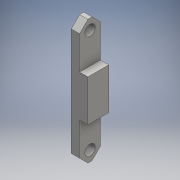
# Autodesk Inventor part: promo_arm2
Saved by Autodesk Inventor 2016 (Build 200138000, 138)
## iProperties
Created: 2016-05-12
Part Number: promo_arm2
Material: 一般
Document SubType Name: Modeling
Designer: 宏太
Density: 1 g/cm^3
Appearance: 既定
Mass: 0.364365 g
Surface Area: 4.86408 cm^2
Volume: 0.364365 cm^3
Author: 宏太
Autodesk Inventor part; units mm, degrees
ref_plane "YZ Plane" through (0, 0, 0) normal (1, 0, 0) x (0, 1, 0)
ref_plane "XZ Plane" through (0, 0, 0) normal (0, 1, 0) x (-1, 0, 0)
ref_plane "XY Plane" through (0, 0, 0) normal (0, 0, 1) x (1, 0, 0)
sketch "スケッチ1" plane through (0, 0, 0) normal (0, 1, 0) x (-1, 0, 0)
  line L0 (-2, -15) -> (2, -15)
  line L1 (2, -15) -> (2, 15)
  line L2 (2, 15) -> (-2, 15)
  line L3 (-2, 15) -> (-2, -15)
  line L4 (-2, -15) -> (2, 15) construction
  line L5 (2, -15) -> (-2, 15) construction
  point P0 (0, 0)
  dimension "d0" = 4
  dimension "d1" = 30
  constraints: 12 end point, 2 midpoint, 2 parallel, 1 horizontal, 1 perpendicular
  measures "d0" distance of L2.end L1.end
  measures "d1" distance of L1.end L0.end
extrude "押し出し1" add sketch "スケッチ1" along normal mid plane 5
sketch "スケッチ2" plane through (0, 2.5, 0) normal (0, 1, 0) x (1, 0, 0)
  line L0 (-2, -15) -> (2, -15) projected
  line L1 (0, -15) -> (2, -15)
  line L2 (2, -15) -> (2, -5)
  line L3 (2, -5) -> (0, -5)
  line L4 (0, -5) -> (0, -15)
  point P0 (0, 0)
  dimension "d4" = 2
  dimension "d5" = 10
  constraints: 8 end point, 2 parallel, 1 horizontal, 1 midpoint, 1 perpendicular
  measures "d4" distance of L3.end L2.end
  measures "d5" distance of L2.end L1.end
extrude "押し出し2" cut sketch "スケッチ2" against normal blind 5
sketch "スケッチ4" plane through (0, 2.5, 15) normal (1, 0, 0) x (0, 0, -1)
  circle A0 centre (2.5, -2.5) radius 1.25
  point P0 (15, -2.5)
  dimension "d12" = 2.5
  constraints: 1 centre point
  measures "d12" diameter of A0
extrude "押し出し4" cut sketch "スケッチ4" against normal blind 5
ref_plane "作業平面1" through (0, 2.5, -15) normal (-1, 0, 0) x (0, 0, 1)
sketch "スケッチ5" plane through (0, 2.5, -15) normal (-1, 0, 0) x (0, 0, 1)
  circle A0 centre (2.5, -2.5) radius 1.25
  point P0 (15, -2.5)
  dimension "d15" = 2.5
  constraints: 1 centre point
  measures "d15" diameter of A0
extrude "押し出し5" cut sketch "スケッチ5" along normal mid plane 5
chamfer "面取り1" distance 2 angle 45 1 edges at (-1, -2.5, 15)
chamfer "面取り2" distance 2 angle 45 1 edges at (-1, 2.5, 15)
chamfer "面取り3" distance 2 angle 45 1 edges at (0, -2.5, -15)
chamfer "面取り4" distance 2 angle 45 1 edges at (0, 2.5, -15)
sketch "スケッチ6" plane through (0, 2.5, -15) normal (-1, 0, 0) x (0, 0, 1)
  line L0 (28, -5) -> (2, -5) projected
  line L1 (0, 0) -> (10, 0)
  line L2 (10, 0) -> (10, -5)
  line L3 (10, -5) -> (0, -5)
  line L4 (0, -5) -> (0, 0)
  point P0 (15, -2.5)
  dimension "d30" = 10
  constraints: 8 end point, 2 parallel, 1 horizontal, 1 perpendicular, 1 point on line
  measures "d30" distance of L2.end L3.end
extrude "押し出し6" cut sketch "スケッチ6" against normal blind 10
